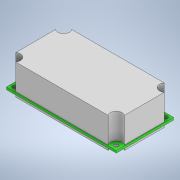
# Autodesk Inventor part: netzteil_3.3V
Saved by Autodesk Inventor 2021 (Build 250183000, 183)
## iProperties
Created: 2021-07-14
Part Number: netzteil_3.3V
Material: Generisch
Document SubType Name: Modeling
Designer: Simon
Density: 1 g/cm^3
Appearance: Vorgabe
Author: Simon
Autodesk Inventor part; units mm, degrees
ref_plane "YZ Plane" through (0, 0, 0) normal (1, 0, 0) x (0, 1, 0)
ref_plane "XZ Plane" through (0, 0, 0) normal (0, 1, 0) x (-1, 0, 0)
ref_plane "XY Plane" through (0, 0, 0) normal (0, 0, 1) x (1, 0, 0)
sketch "Skizze1" plane through (0, 0, 0) normal (0, 1, 0) x (-1, 0, 0)
  line L0 (47, -24.5) -> (-47, -24.5)
  line L1 (-47, -24.5) -> (-47, 24.5)
  line L2 (-47, 24.5) -> (47, 24.5)
  line L3 (47, 24.5) -> (47, -24.5)
  point P0 (0, 0)
  point P1 (0, -24.5)
  point P2 (47, 0)
  dimension "d0" = 49
  dimension "d1" = 94
  constraints: 8 end point, 2 midpoint, 2 parallel, 1 horizontal, 1 horizontal alignment, 1 perpendicular, 1 vertical alignment
  measures "d0" distance between parallel lines of L2 L0
  measures "d1" distance between parallel lines of L3 L1
extrude "Extrusion1" add sketch "Skizze1" along normal blind 2
sketch "Skizze2" plane through (0, 2, 0) normal (0, 1, 0) x (1, 0, 0)
  circle A0 centre (-43.5, 21) radius 1.75
  circle A1 centre (-43.5, -21) radius 1.75
  circle A2 centre (43.5, -21) radius 1.75
  circle A3 centre (43.5, 21) radius 1.75
  point P0 (0, 0)
  dimension "d4" = 3.5
  dimension "d5" = 3.5
  dimension "d6" = 3.5
  dimension "d7" = 3.5
  dimension "d8" = 87
  dimension "d9" = 43.5
  dimension "d10" = 42
  dimension "d11" = 21
  constraints: 4 centre point, 2 horizontal alignment, 2 vertical alignment
  measures "d4" diameter of A0
  measures "d5" diameter of A1
  measures "d6" diameter of A2
  measures "d7" diameter of A3
  measures "d8" distance of A3.centre A0.centre
  measures "d9" horizontal distance of point (0, 0) A0.centre
  measures "d10" distance of A1.centre A0.centre
  measures "d11" vertical distance of A0.centre point (0, 0)
extrude "Extrusion2" cut sketch "Skizze2" against normal through all
sketch "Skizze4" plane through (0, 2, 0) normal (0, 1, 0) x (1, 0, 0)
  line L0 (-39.5, 24) -> (39.5, 24)
  line L1 (46.5, 17) -> (46.5, -17)
  line L2 (39.5, -24) -> (-39.5, -24)
  line L3 (-46.5, -17) -> (-46.5, 17)
  line L4 (47, -24.5) -> (47, 24.5) projected
  line L5 (47, 24.5) -> (-47, 24.5) projected
  line L6 (-47, -24.5) -> (47, -24.5) projected
  line L7 (-47, 24.5) -> (-47, -24.5) projected
  circle A0 centre (-43.5, 21) radius 1.75 projected
  arc A1 (-46.5, 17) -> (-39.5, 24) centre (-43.5, 21) ccw
  circle A2 centre (-43.5, -21) radius 1.75 projected
  arc A3 (-39.5, -24) -> (-46.5, -17) centre (-43.5, -21) ccw
  circle A4 centre (43.5, -21) radius 1.75 projected
  arc A5 (46.5, -17) -> (39.5, -24) centre (43.5, -21) ccw
  arc A6 (39.5, 24) -> (46.5, 17) centre (43.5, 21) ccw
  circle A7 centre (43.5, 21) radius 1.75 projected
  point P0 (0, 0)
  dimension "d14" = 0.5
  dimension "d15" = 0.5
  dimension "d16" = 0.5
  dimension "d17" = 0.5
  dimension "d19" = 5
  dimension "d20" = 5
  dimension "d21" = 5
  dimension "d22" = 5
  constraints: 9 point on circle, 8 end point, 4 centre point, 4 coincident, 2 parallel, 1 horizontal, 1 perpendicular
  measures "d14" distance between parallel lines of L4 L1
  measures "d15" distance between parallel lines of L5 L0
  measures "d16" distance between parallel lines of L6 L2
  measures "d17" distance between parallel lines of L7 L3
  measures "d19" radius of A6
  measures "d20" radius of A1
  measures "d21" radius of A5
  measures "d22" radius of A3
extrude "Extrusion3" add sketch "Skizze4" along normal blind 22 and the other way blind 4 contours L0 A6 L1 A5 L2 A3 L3 A1
equation "\"d9\" = 0.5 * d8"
equation "\"d11\" = 0.5 * d10"
equation "\"d14\" = d15"
equation "\"d16\" = d15"
equation "\"d17\" = d15"
equation "\"d19\" = d20"
equation "\"d21\" = d20"
equation "\"d22\" = d20"
